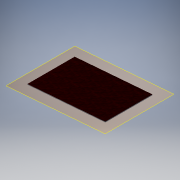
# Autodesk Inventor part: Dach
Saved by Autodesk Inventor 2017 (Build 210142000, 142)
## iProperties
Created: 2017-05-11
Part Number: Dach
Material: Generic
Document SubType Name: Modeling
Designer: Fake
Density: 1 g/cm^3
Appearance: Default
Author: Fake
Autodesk Inventor part; units mm, degrees
ref_plane "YZ Plane" through (0, 0, 0) normal (1, 0, 0) x (0, 1, 0)
ref_plane "XZ Plane" through (0, 0, 0) normal (0, 1, 0) x (-1, 0, 0)
ref_plane "XY Plane" through (0, 0, 0) normal (0, 0, 1) x (1, 0, 0)
ref_plane "Arbeitsebene1" through (3246.2358, -2250, 2559.6989) normal (-0.0797452, 0, 0.9968153) x (0, -1, 0)
sketch "Skizze1" plane through (3246.2358, -2250, 2559.6989) normal (-0.0797452, 0, 0.9968153) x (0, -1, 0)
  line L0 (-850, -848.9395) -> (-3650, -848.9395) projected
  line L1 (-850, -5664.275) -> (-850, -848.9395) projected
  line L2 (-3650, -5664.275) -> (-850, -5664.275) projected
  line L3 (-3650, -848.9395) -> (-3650, -5664.275) projected
  line L4 (-3750, -5764.5945) -> (-3750, -748.62) projected
  line L5 (-750, -5764.5945) -> (-3750, -5764.5945) projected
  line L6 (-750, -748.62) -> (-750, -5764.5945) projected
  line L7 (-750, -748.62) -> (-3750, -748.62) projected
  line L8 (-3950, -6064.5945) -> (-550, -6064.5945)
  line L9 (-550, -6064.5945) -> (-550, -448.62)
  line L10 (-550, -448.62) -> (-3950, -448.62)
  line L11 (-3950, -448.62) -> (-3950, -6064.5945)
  dimension "d0" = 200
  dimension "d1" = 300
  dimension "d2" = 300
  dimension "d3" = 200
  constraints: 8 end point, 2 parallel, 1 horizontal, 1 perpendicular
  measures "d0" distance between parallel lines of L11 L4
  measures "d1" distance between parallel lines of L7 L10
  measures "d2" distance between parallel lines of L5 L8
  measures "d3" distance between parallel lines of L6 L9
extrude "Extrusion1" add sketch "Skizze1" along normal blind 50 contours L1 L2 L3 L0 | L4 L7 L6 L5 | L11 L10 L9 L8
equation "\"d2\" = d1"
equation "\"d3\" = d0"
